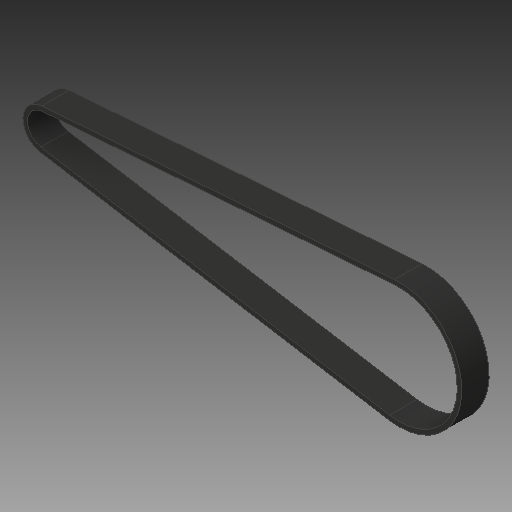
# Autodesk Inventor part: Belt
Saved by Autodesk Inventor 2018.2 (Build 222227000, 227)
## iProperties
Created: 2018-03-07
Part Number: Belt
Material: Generic
Document SubType Name: Modeling
Designer: Moochster
Density: 1 g/cm^3
Appearance: Rubber - Black
Mass: 1.27078 g
Surface Area: 29.6514 cm^2
Volume: 1.27078 cm^3
Author: Moochster
Autodesk Inventor part; units mm, degrees
ref_plane "YZ Plane" through (0, 0, 0) normal (1, 0, 0) x (0, 1, 0)
ref_plane "XZ Plane" through (0, 0, 0) normal (0, 1, 0) x (-1, 0, 0)
ref_plane "XY Plane" through (0, 0, 0) normal (0, 0, 1) x (1, 0, 0)
sketch "Sketch1" plane through (0, 0, 0) normal (0, 0, 1) x (1, 0, 0)
  circle A0 centre (66.3829, 0.6317) radius 13.7761 projected
  line L0 (-12.0738, 8.6506) -> (65.3682, 14.3704)
  line L1 (-12.4772, -0.2842) -> (64.1342, -12.9596)
  line L2 (-12.0001, 7.6533) -> (-8.9346, 7.8797)
  arc A1 (64.2974, -11.973) -> (65.4418, 13.3731) centre (66.3829, 0.6317) ccw
  line L3 (64.2974, -11.973) -> (59.2137, -11.1319)
  arc A2 (-12.0001, 7.6533) -> (-12.314, 0.7024) centre (-11.7421, 4.1591) ccw
  line L4 (3.1814, -1.8614) -> (-12.314, 0.7024)
  line L5 (-8.9346, 7.8797) -> (60.3029, 12.9936)
  line L6 (59.2137, -11.1319) -> (3.1814, -1.8614)
  line L7 (60.3029, 12.9936) -> (65.4418, 13.3731)
  arc A3 (-9.1781, 7.8617) -> (-9.5222, 0.2405) centre (-11.7421, 4.1591) ccw
  arc A4 (-9.5222, 0.2405) -> (-9.1781, 7.8617) centre (-11.7421, 4.1591) ccw
  point P0 (0, 0)
  dimension "d0" = 1
  constraints: 16 end point, 16 tangent, 14 point on circle, 4 centre point, 2 concentric, 2 point on line, 2 other
  measures "d0" distance between parallel lines of L1 L3
extrude "Extrusion2" add sketch "Sketch1" along normal blind 6 contours A0 L3 A1 L7 | A0 L5 L2 A3 L0 | L1 A3 L4 L6 A0 | A3 L2 A2 L4 picked at (66.3473, -12.7206)
body "Solid2"
